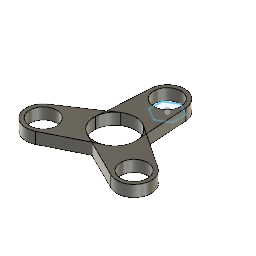
Fidget_Spinner (Autodesk Fusion 360 design; units mm, degrees)
Autodesk Fusion 360 part; units mm, degrees
sketch "Sketch1" plane through (0, 0, 0) normal (0, 0, 1) x (1, 0, 0)
  circle A0 centre (0, 0) radius 11
  circle A1 centre (0, 28) radius 7.19
  circle A2 centre (0, 28) radius 9.25
  line L0 (-10.9785, 0.6875) -> (-9.2319, 28.5781)
  line L1 (10.9785, 0.6875) -> (9.2319, 28.5781)
  dimension "d1" = 22
  dimension "d3" = 14.38
  dimension "d5" = 18.5
  constraint coincident A0.centre origin
  constraint concentric A1 A2
  constraint coincident A0 L0.start
  constraint coincident A2 L0.end
  constraint tangent A2 L0
  constraint tangent A0 L0
  constraint coincident A0 L1.start
  constraint coincident A2 L1.end
  constraint tangent A2 L1
  constraint tangent A0 L1
  measures "d1" diameter of A0
  measures "d3" diameter of A1
  measures "d5" diameter of A2
sketch "Sketch3" plane through (0, 0, 0) normal (0, 0, 1) x (1, 0, 0)
  line L0 (-0.0645, 35.1897) -> (-6.2587, 31.539)
  line L1 (-6.2587, 31.539) -> (-6.1942, 24.3493)
  line L2 (-6.1942, 24.3493) -> (0.0645, 20.8103)
  line L3 (0.0645, 20.8103) -> (6.2587, 24.461)
  line L4 (6.2587, 24.461) -> (6.1942, 31.6507)
  line L5 (6.1942, 31.6507) -> (-0.0645, 35.1897)
  point P0 (0, 28)
  dimension "d7" = 7.19
  measures "d7" distance of L0.start P0
extrude "Extrude1" add sketch "Sketch1" along normal blind 6.15 contours A0 A2 L0 L1 | A2 makes body 1
pattern_circular "C-Pattern1" count 3 over 360 about axis through (0, 0, 1.75) along (0, 0, 1) of bodies 1 makes body 2 at (-13.2292, -17.0879, 0) makes body 3 at (21.4131, -2.9129, 0)
sketch "Sketch2" plane through (0, 0, 0) normal (0, 0, 1) x (1, 0, 0)
  line L0 (6.1908, 38.6565) -> (-0.0712, 42.1896)
  line L1 (-0.0712, 42.1896) -> (-6.262, 38.5331)
  line L2 (-6.262, 38.5331) -> (-6.1908, 31.3435)
  line L3 (-6.1908, 31.3435) -> (0.0712, 27.8104)
  line L4 (0.0712, 27.8104) -> (6.262, 31.4669)
  line L5 (6.262, 31.4669) -> (6.1908, 38.6565)
  point P0 (0, 35)
  dimension "d6" = 7.19
  measures "d6" distance of L0.start P0
